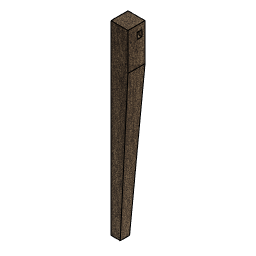
Leg (Autodesk Fusion 360 design; units mm, degrees)
Autodesk Fusion 360 part; units mm, degrees
sketch "Sketch2" plane through (0, 0, 0) normal (0, 0, 1) x (1, 0, 0)
  line L0 (-34.925, 34.925) -> (34.925, 34.925)
  line L1 (34.925, 34.925) -> (34.925, -34.925)
  line L2 (34.925, -34.925) -> (-34.925, -34.925)
  line L3 (-34.925, -34.925) -> (-34.925, 34.925)
  line L4 (-34.925, 34.925) -> (34.925, -34.925) construction
  line L5 (34.925, 34.925) -> (-34.925, -34.925) construction
  dimension "d1" = 69.85
  dimension "d2" = 69.85
  constraint horizontal L0
  constraint perpendicular L0 L1
  constraint parallel L0 L2
  constraint parallel L1 L3
  constraint coincident L4 origin
  constraint coincident L5 origin
  measures "d1" distance of L1.end L2.end
  measures "d2" distance of L0.end L1.end
extrude "Extrude1" add sketch "Sketch2" along normal blind 762
chamfer "Chamfer1" distance 31.75 distance2 609.6 2 edges at (34.925, 0, 0) (0, 34.925, 0) measured on face at (11.6417, -11.6417, 0) measured on face at (11.6417, -11.6417, 0)
sketch "Sketch6" plane through (34.925, 0, 0) normal (1, 0, 0) x (0, 1, 0)
  line L0 (-34.925, 609.6) -> (34.925, 609.6)
  line L1 (34.925, 609.6) -> (34.925, 762)
  line L2 (34.925, 762) -> (-34.925, 762)
  line L3 (-34.925, 762) -> (-34.925, 609.6)
  line L4 (-34.925, 762) -> (-34.925, 723.9) construction
  line L5 (-34.925, 723.9) -> (12.7, 723.9) construction
  line L6 (3.175, 736.6) -> (22.225, 736.6)
  line L7 (22.225, 736.6) -> (22.225, 711.2)
  line L8 (22.225, 711.2) -> (3.175, 711.2)
  line L9 (3.175, 711.2) -> (3.175, 736.6)
  line L10 (3.175, 736.6) -> (22.225, 711.2) construction
  line L11 (22.225, 736.6) -> (3.175, 711.2) construction
  point P0 (12.7, 723.9)
  dimension "d23" = 38.1
  dimension "d24" = 47.625
  dimension "d25" = 19.05
  dimension "d26" = 25.4
  constraint coincident L2.end L3.start
  constraint perpendicular L0 L4
  constraint perpendicular L4 L5
  constraint horizontal L6
  constraint perpendicular L6 L7
  constraint parallel L6 L8
  constraint parallel L7 L9
  constraint coincident L10 P0
  constraint coincident L11 P0
  constraint coincident P0 L5.end
  measures "d23" distance of L2.end L4.end
  measures "d24" distance of L4.end P0
  measures "d25" distance of L7.end L8.end
  measures "d26" distance of L6.end L7.end
extrude "Extrude5" cut sketch "Sketch6" against normal blind 31.75 contours L6 L7 L8 L9
sketch "Sketch7" plane through (0, 34.925, 0) normal (0, 1, 0) x (-1, 0, 0)
  line L0 (-34.925, 609.6) -> (34.925, 609.6)
  line L1 (34.925, 609.6) -> (34.925, 762)
  line L2 (34.925, 762) -> (-34.925, 762)
  line L3 (-34.925, 762) -> (-34.925, 609.6)
  line L4 (34.925, 762) -> (34.925, 723.9) construction
  line L5 (34.925, 723.9) -> (-12.7, 723.9) construction
  line L6 (-22.225, 736.6) -> (-3.175, 736.6)
  line L7 (-3.175, 736.6) -> (-3.175, 711.2)
  line L8 (-3.175, 711.2) -> (-22.225, 711.2)
  line L9 (-22.225, 711.2) -> (-22.225, 736.6)
  line L10 (-22.225, 736.6) -> (-3.175, 711.2) construction
  line L11 (-3.175, 736.6) -> (-22.225, 711.2) construction
  point P0 (-12.7, 723.9)
  dimension "d29" = 38.1
  dimension "d30" = 47.625
  dimension "d31" = 19.05
  dimension "d32" = 25.4
  constraint coincident L1.end L2.start
  constraint perpendicular L2 L4
  constraint perpendicular L1 L5
  constraint horizontal L6
  constraint perpendicular L6 L7
  constraint parallel L6 L8
  constraint parallel L7 L9
  constraint coincident L10 P0
  constraint coincident L11 P0
  constraint coincident P0 L5.end
  measures "d29" distance of L1.end L4.end
  measures "d30" distance of L4.end P0
  measures "d31" distance of L7.end L8.end
  measures "d32" distance of L6.end L7.end
extrude "Extrude6" cut sketch "Sketch7" against normal blind 31.75 contours L6 L7 L8 L9
equation "d24 = 1.125 in + 0.375 in + 0.375 in"
